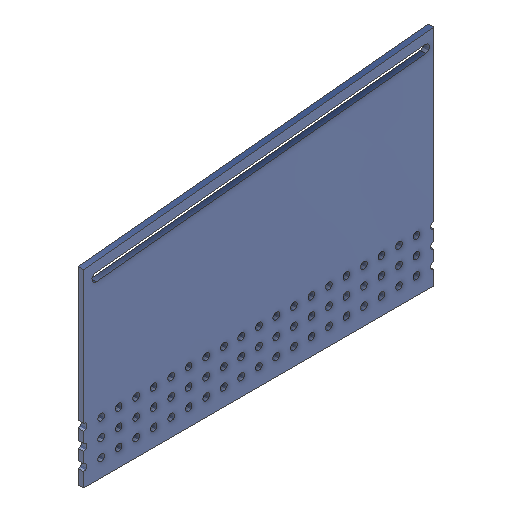
# Autodesk Inventor part: Guia - Intake
Saved by Autodesk Inventor 2025.3 (Build 293356000, 356)
## iProperties
Created: 2026-05-13
Part Number: Guia - Intake
Material: Genérico
Document SubType Name: Modeling
Designer: djair.oliveira
Density: 1 g/cm^3
Appearance: Padrão
Author: djair.oliveira
Autodesk Inventor part; units mm, degrees
ref_plane "YZ Plane" through (0, 0, 0) normal (1, 0, 0) x (0, 1, 0)
ref_plane "XZ Plane" through (0, 0, 0) normal (0, 1, 0) x (-1, 0, 0)
ref_plane "XY Plane" through (0, 0, 0) normal (0, 0, 1) x (1, 0, 0)
sketch "Esboço1" plane through (0, 0, 0) normal (1, 0, 0) x (0, 1, 0)
  line L0 (0, 0) -> (127, 0)
  line L1 (127, 0) -> (152.4, -254)
  line L2 (152.4, -254) -> (0, -254)
  line L3 (0, -254) -> (0, 0)
  circle A0 centre (12.7, 0) radius 2.5
  circle A1 centre (25.4, 0) radius 2.5
  circle A2 centre (38.1, 0) radius 2.5
  circle A3 centre (38.1, -12.7) radius 2.5
  circle A4 centre (25.4, -12.7) radius 2.5
  circle A5 centre (12.7, -12.7) radius 2.5
  circle A6 centre (38.1, -25.4) radius 2.5
  circle A7 centre (25.4, -25.4) radius 2.5
  circle A8 centre (12.7, -25.4) radius 2.5
  circle A9 centre (38.1, -38.1) radius 2.5
  circle A10 centre (25.4, -38.1) radius 2.5
  circle A11 centre (12.7, -38.1) radius 2.5
  circle A12 centre (38.1, -50.8) radius 2.5
  circle A13 centre (25.4, -50.8) radius 2.5
  circle A14 centre (12.7, -50.8) radius 2.5
  circle A15 centre (38.1, -63.5) radius 2.5
  circle A16 centre (25.4, -63.5) radius 2.5
  circle A17 centre (12.7, -63.5) radius 2.5
  circle A18 centre (38.1, -76.2) radius 2.5
  circle A19 centre (25.4, -76.2) radius 2.5
  circle A20 centre (12.7, -76.2) radius 2.5
  circle A21 centre (38.1, -88.9) radius 2.5
  circle A22 centre (25.4, -88.9) radius 2.5
  circle A23 centre (12.7, -88.9) radius 2.5
  circle A24 centre (38.1, -101.6) radius 2.5
  circle A25 centre (25.4, -101.6) radius 2.5
  circle A26 centre (12.7, -101.6) radius 2.5
  circle A27 centre (38.1, -114.3) radius 2.5
  circle A28 centre (25.4, -114.3) radius 2.5
  circle A29 centre (12.7, -114.3) radius 2.5
  circle A30 centre (38.1, -127) radius 2.5
  circle A31 centre (25.4, -127) radius 2.5
  circle A32 centre (12.7, -127) radius 2.5
  circle A33 centre (38.1, -139.7) radius 2.5
  circle A34 centre (25.4, -139.7) radius 2.5
  circle A35 centre (12.7, -139.7) radius 2.5
  circle A36 centre (38.1, -152.4) radius 2.5
  circle A37 centre (25.4, -152.4) radius 2.5
  circle A38 centre (12.7, -152.4) radius 2.5
  circle A39 centre (38.1, -165.1) radius 2.5
  circle A40 centre (25.4, -165.1) radius 2.5
  circle A41 centre (12.7, -165.1) radius 2.5
  circle A42 centre (38.1, -177.8) radius 2.5
  circle A43 centre (25.4, -177.8) radius 2.5
  circle A44 centre (12.7, -177.8) radius 2.5
  circle A45 centre (38.1, -190.5) radius 2.5
  circle A46 centre (25.4, -190.5) radius 2.5
  circle A47 centre (12.7, -190.5) radius 2.5
  circle A48 centre (38.1, -203.2) radius 2.5
  circle A49 centre (25.4, -203.2) radius 2.5
  circle A50 centre (12.7, -203.2) radius 2.5
  circle A51 centre (38.1, -215.9) radius 2.5
  circle A52 centre (25.4, -215.9) radius 2.5
  circle A53 centre (12.7, -215.9) radius 2.5
  circle A54 centre (38.1, -228.6) radius 2.5
  circle A55 centre (25.4, -228.6) radius 2.5
  circle A56 centre (12.7, -228.6) radius 2.5
  circle A57 centre (38.1, -241.3) radius 2.5
  circle A58 centre (25.4, -241.3) radius 2.5
  circle A59 centre (12.7, -241.3) radius 2.5
  circle A60 centre (38.1, -254) radius 2.5
  circle A61 centre (25.4, -254) radius 2.5
  circle A62 centre (12.7, -254) radius 2.5
  circle A63 centre (127.2985, -2.9851) radius 3
  circle A64 centre (127.8955, -8.9553) radius 3
  circle A65 centre (128.4926, -14.9256) radius 3
  circle A66 centre (129.0896, -20.8958) radius 3
  circle A67 centre (129.6866, -26.866) radius 3
  circle A68 centre (130.2836, -32.8362) radius 3
  circle A69 centre (130.8806, -38.8065) radius 3
  circle A70 centre (131.4777, -44.7767) radius 3
  circle A71 centre (132.0747, -50.7469) radius 3
  circle A72 centre (132.6717, -56.7171) radius 3
  circle A73 centre (133.2687, -62.6873) radius 3
  circle A74 centre (133.8658, -68.6576) radius 3
  circle A75 centre (134.4628, -74.6278) radius 3
  circle A76 centre (135.0598, -80.598) radius 3
  circle A77 centre (135.6568, -86.5682) radius 3
  circle A78 centre (136.2538, -92.5385) radius 3
  circle A79 centre (136.8509, -98.5087) radius 3
  circle A80 centre (137.4479, -104.4789) radius 3
  circle A81 centre (138.0449, -110.4491) radius 3
  circle A82 centre (138.6419, -116.4194) radius 3
  circle A83 centre (139.239, -122.3896) radius 3
  circle A84 centre (139.836, -128.3598) radius 3
  circle A85 centre (140.433, -134.33) radius 3
  circle A86 centre (141.03, -140.3002) radius 3
  circle A87 centre (141.627, -146.2705) radius 3
  circle A88 centre (142.2241, -152.2407) radius 3
  circle A89 centre (142.8211, -158.2109) radius 3
  circle A90 centre (143.4181, -164.1811) radius 3
  circle A91 centre (144.0151, -170.1514) radius 3
  circle A92 centre (144.6122, -176.1216) radius 3
  circle A93 centre (145.2092, -182.0918) radius 3
  circle A94 centre (145.8062, -188.062) radius 3
  circle A95 centre (146.4032, -194.0323) radius 3
  circle A96 centre (147.0002, -200.0025) radius 3
  circle A97 centre (147.5973, -205.9727) radius 3
  circle A98 centre (148.1943, -211.9429) radius 3
  circle A99 centre (148.7913, -217.9131) radius 3
  circle A100 centre (149.3883, -223.8834) radius 3
  circle A101 centre (149.9854, -229.8536) radius 3
  circle A102 centre (150.5824, -235.8238) radius 3
  circle A103 centre (151.1794, -241.794) radius 3
  circle A104 centre (151.7764, -247.7643) radius 3
  circle A105 centre (152.3734, -253.7345) radius 3
  line L4 (127, 0) -> (137.0499, 0)
  line L5 (137.0499, 0) -> (162.4499, -254)
  line L6 (162.4499, -254) -> (152.4, -254)
  line L7 (151.7764, -247.7643) -> (127.8955, -8.9553) construction
  line L8 (154.7615, -247.4657) -> (130.8806, -8.6568)
  line L9 (124.9104, -9.2538) -> (148.7913, -248.0628)
  arc A106 (148.7913, -248.0628) -> (154.7615, -247.4657) centre (151.7764, -247.7643) ccw
  arc A107 (130.8806, -8.6568) -> (124.9104, -9.2538) centre (127.8955, -8.9553) ccw
  point P0 (40.6, 0)
  point P1 (35.6, 0)
  point P2 (27.9, 0)
  point P3 (22.9, 0)
  point P4 (15.2, 0)
  point P5 (10.2, 0)
  point P6 (10.2, -254)
  point P7 (15.2, -254)
  point P8 (22.9, -254)
  point P9 (27.9, -254)
  point P10 (35.6, -254)
  point P11 (40.6, -254)
  point P12 (127.597, -5.9702)
  point P13 (128.194, -11.9404)
  point P14 (128.7911, -17.9107)
  point P15 (129.3881, -23.8809)
  point P16 (129.9851, -29.8511)
  point P17 (130.5821, -35.8213)
  point P18 (131.1792, -41.7916)
  point P19 (131.7762, -47.7618)
  point P20 (132.3732, -53.732)
  point P21 (132.9702, -59.7022)
  point P22 (133.5672, -65.6725)
  point P23 (134.1643, -71.6427)
  point P24 (134.7613, -77.6129)
  point P25 (135.3583, -83.5831)
  point P26 (135.9553, -89.5533)
  point P27 (136.5524, -95.5236)
  point P28 (137.1494, -101.4938)
  point P29 (137.7464, -107.464)
  point P30 (138.3434, -113.4342)
  point P31 (138.9404, -119.4045)
  point P32 (139.5375, -125.3747)
  point P33 (140.1345, -131.3449)
  point P34 (140.7315, -137.3151)
  point P35 (141.3285, -143.2854)
  point P36 (141.9256, -149.2556)
  point P37 (142.5226, -155.2258)
  point P38 (143.1196, -161.196)
  point P39 (143.7166, -167.1662)
  point P40 (144.3136, -173.1365)
  point P41 (144.9107, -179.1067)
  point P42 (145.5077, -185.0769)
  point P43 (146.1047, -191.0471)
  point P44 (146.7017, -197.0174)
  point P45 (147.2988, -202.9876)
  point P46 (147.8958, -208.9578)
  point P47 (148.4928, -214.928)
  point P48 (149.0898, -220.8983)
  point P49 (149.6868, -226.8685)
  point P50 (150.2839, -232.8387)
  point P51 (150.8809, -238.8089)
  point P52 (151.4779, -244.7791)
  point P53 (152.0749, -250.7494)
  point P54 (152.0749, -250.7494)
  point P55 (151.4779, -244.7791)
  point P56 (150.8809, -238.8089)
  point P57 (150.2839, -232.8387)
  point P58 (149.6868, -226.8685)
  point P59 (149.0898, -220.8983)
  point P60 (148.4928, -214.928)
  point P61 (147.8958, -208.9578)
  point P62 (147.2988, -202.9876)
  point P63 (146.7017, -197.0174)
  point P64 (146.1047, -191.0471)
  point P65 (145.5077, -185.0769)
  point P66 (144.9107, -179.1067)
  point P67 (144.3136, -173.1365)
  point P68 (143.7166, -167.1662)
  point P69 (143.1196, -161.196)
  point P70 (142.5226, -155.2258)
  point P71 (141.9256, -149.2556)
  point P72 (141.3285, -143.2854)
  point P73 (140.7315, -137.3151)
  point P74 (140.1345, -131.3449)
  point P75 (139.5375, -125.3747)
  point P76 (138.9404, -119.4045)
  point P77 (138.3434, -113.4342)
  point P78 (137.7464, -107.464)
  point P79 (137.1494, -101.4938)
  point P80 (136.5524, -95.5236)
  point P81 (135.9553, -89.5533)
  point P82 (135.3583, -83.5831)
  point P83 (134.7613, -77.6129)
  point P84 (134.1643, -71.6427)
  point P85 (133.5672, -65.6725)
  point P86 (132.9702, -59.7022)
  point P87 (132.3732, -53.732)
  point P88 (131.7762, -47.7618)
  point P89 (131.1792, -41.7916)
  point P90 (130.5821, -35.8213)
  point P91 (129.9851, -29.8511)
  point P92 (129.3881, -23.8809)
  point P93 (128.7911, -17.9107)
  point P94 (128.194, -11.9404)
  point P95 (127.597, -5.9702)
  point P96 (139.836, -128.3598)
  point P97 (130.8806, -8.6568)
  point P98 (148.7913, -248.0628)
  dimension "d16" = 6
  dimension "d0" = 254
  dimension "d1" = 152.4
  dimension "d2" = 127
  dimension "d3" = 5
  dimension "d4" = 12.7
  dimension "d5" = 12.7
  dimension "d6" = 12.7
  dimension "d9" = 12.7
  dimension "d19" = 6
  dimension "d26" = 252
  dimension "d27" = 10
  constraints: 65 centre point, 20 end point, 4 point on circle, 4 tangent, 3 point on line, 2 equal radius, 2 horizontal, 2 parallel, 1 collinear, 1 midpoint, 1 perpendicular, 1 vertical, 340 other
  measures "d0" distance of L2.end L0.start
  measures "d1" distance of L2.start L2.end
  measures "d2" distance of L0.start L0.end
  measures "d3" diameter of A2
  measures "d4" distance of A1.centre A2.centre
  measures "d5" distance of A1.centre A0.centre
  measures "d6" distance from line of L3 A0.centre
  measures "d9" distance of A2.centre A3.centre
  measures "d19" distance of point (127.299, -2.985) L7.end
  measures "d26" distance of point (152.373, -253.734) point (127.299, -2.985)
  measures "d27" distance from line of point (152.075, -250.749) L5
extrude "Extrusão1" add sketch "Esboço1" along normal blind 4 contours L0 A63 A64 L9 A104 A105 L2 A60 A61 A62 L3 A0 A1 A2 | L4 A63 L1 | L1 A63 | A63 L4 L5 L6 A105 A104 L8 A64 | L6 L1 A105 | A105 L1 L2
equation "\"d5\" = d4"
